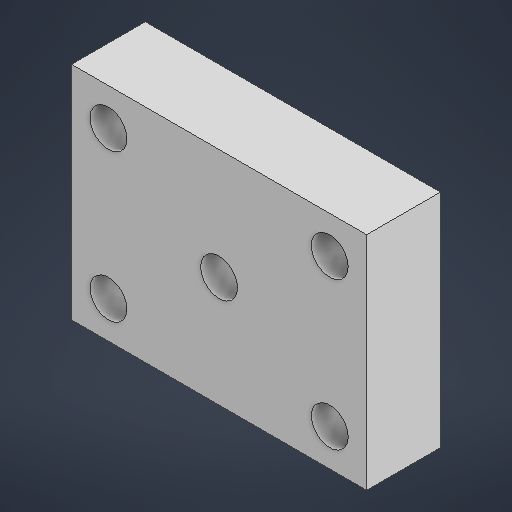
# Autodesk Inventor part: center block
Saved by Autodesk Inventor 2026.1 (Build 301233000, 233)
## iProperties
Created: 2026-06-10
Part Number: center block
Material: Generic
Document SubType Name: Modeling
Designer: share
Density: 1 g/cm^3
Appearance: Default
Author: share
Autodesk Inventor part; units mm, degrees
ref_plane "YZ Plane" through (0, 0, 0) normal (1, 0, 0) x (0, 1, 0)
ref_plane "XZ Plane" through (0, 0, 0) normal (0, 1, 0) x (-1, 0, 0)
ref_plane "XY Plane" through (0, 0, 0) normal (0, 0, 1) x (1, 0, 0)
sketch "Sketch1" plane through (0, 0, 0) normal (0, 0, 1) x (1, 0, 0)
  line L0 (-50.8, -38.1) -> (50.8, -38.1)
  line L1 (50.8, -38.1) -> (50.8, 38.1)
  line L2 (50.8, 38.1) -> (-50.8, 38.1)
  line L3 (-50.8, 38.1) -> (-50.8, -38.1)
  line L4 (-50.8, -38.1) -> (50.8, 38.1) construction
  line L5 (50.8, -38.1) -> (-50.8, 38.1) construction
  line L6 (-38.1, -25.4) -> (38.1, -25.4)
  line L7 (38.1, -25.4) -> (38.1, 25.4)
  line L8 (38.1, 25.4) -> (-38.1, 25.4)
  line L9 (-38.1, 25.4) -> (-38.1, -25.4)
  line L10 (-38.1, -25.4) -> (38.1, 25.4) construction
  line L11 (38.1, -25.4) -> (-38.1, 25.4) construction
  circle A0 centre (-38.1, 25.4) radius 6.35
  circle A1 centre (38.1, 25.4) radius 6.35
  circle A2 centre (-38.1, -25.4) radius 6.35
  circle A3 centre (38.1, -25.4) radius 6.35
  circle A4 centre (0, 0) radius 6.35
  dimension "d0" = 101.6
  dimension "d1" = 76.2
  dimension "d2" = 76.2
  dimension "d3" = 50.8
  dimension "d4" = 12.7
  constraints: 24 end point, 5 centre point, 5 coincident, 4 equal radius, 4 midpoint, 4 parallel, 2 horizontal, 2 perpendicular
  measures "d0" distance between parallel lines of L1 L3
  measures "d1" distance between parallel lines of L0 L2
  measures "d2" distance between parallel lines of L7 L9
  measures "d3" distance between parallel lines of L6 L8
  measures "d4" diameter of A0
extrude "Extrusion1" add sketch "Sketch1" along normal blind 25.4 contours L3 L2 L1 L0 | A2 L9 A0 L8 A1 L7 A3 L6
body "Solid1"
